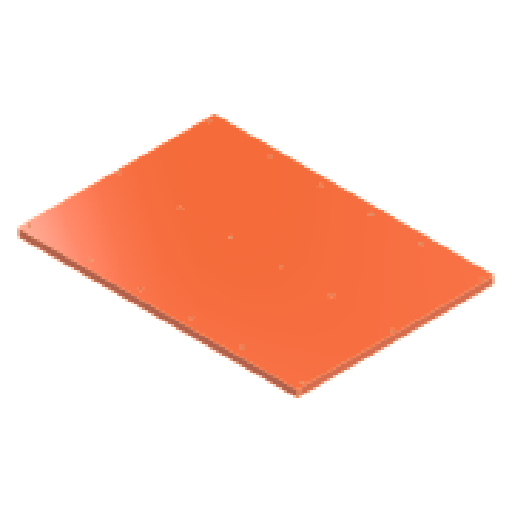
# Autodesk Inventor part: GRJ-04-101A
Saved by Autodesk Inventor 2026.1 (Build 301233000, 233)
## iProperties
Company: Gree
Created: 2025-09-10
Part Number: GRJ-04-101A
Material: Fenolite OR
Document SubType Name: Modeling
Designer: Willian Pinheiro
Density: 1.38 g/cm^3
Appearance: Suave - Laranja claro
Project: GRJ-04
Checked By: Antonio Lucas
Engr Approved By: Antonio Lucas
Description: Base Principal A
Mfg Approved By: Anderson Oliveira
Mass: 1474.18 g
Surface Area: 2294.98 cm^2
Volume: 1068.25 cm^3
Total: 1
Dimensões: 10 x 275 x 390 mm
Author: Willian Pinheiro
Title: Pasta Dissipador G
Revision Number: 00
Autodesk Inventor part; units mm, degrees
ref_plane "YZ Plane" through (0, 0, 0) normal (1, 0, 0) x (0, 1, 0)
ref_plane "XZ Plane" through (0, 0, 0) normal (0, 1, 0) x (-1, 0, 0)
ref_plane "XY Plane" through (0, 0, 0) normal (0, 0, 1) x (1, 0, 0)
sketch "Esboço1" plane through (0, 0, 0) normal (0, 0, 1) x (1, 0, 0)
  line L0 (-195, -137.5) -> (195, -137.5)
  line L1 (195, -137.5) -> (195, 137.5)
  line L2 (195, 137.5) -> (-195, 137.5)
  line L3 (-195, 137.5) -> (-195, -137.5)
  line L4 (190, -137.5) -> (190, 137.5) construction
  line L5 (-273, 0) -> (273, 0) construction
  line L6 (0, -192.5) -> (0, 192.5) construction
  line L7 (-70, 137.5) -> (-70, -137.5) construction
  point P0 (0, 0)
  point P1 (190, 125)
  point P2 (190, 0)
  point P3 (190, -125)
  point P4 (35, 125)
  point P5 (35, 0)
  point P6 (35, -125)
  point P7 (-190, 125)
  point P8 (-190, 0)
  point P9 (-190, -125)
  point P10 (-35, 125)
  point P11 (-35, 0)
  point P12 (-35, -125)
  point P13 (-105, -125)
  point P14 (-105, 0)
  point P15 (-105, 125)
  point P16 (105, 125)
  point P17 (105, 0)
  point P18 (105, -125)
  dimension "d0" = 390
  dimension "d1" = 275
  dimension "d11" = 125
  dimension "d12" = 125
  dimension "d14" = 70
  dimension "d15" = 380
  dimension "d23" = 250
  dimension "d25" = 70
  constraints: 12 end point, 12 symmetric about line, 7 point on line, 3 horizontal alignment, 3 perpendicular, 2 parallel, 2 vertical alignment, 1 horizontal, 1 midpoint, 2 other
  measures "d0" distance of L1.end L2.end
  measures "d1" distance of L2.end L0.start
  measures "d11" distance of point (190, -125) point (190, 0)
  measures "d12" distance of point (190, 125) point (190, 0)
  measures "d14" distance of point (-35, 125) point (35, 125)
  measures "d15" distance of point (-190, 125) point (190, 125)
  measures "d23" distance of point (190, 125) point (190, -125)
  measures "d25" distance of point (-35, 125) point (-105, 125)
extrude "Extrusão1" add sketch "Esboço1" along normal blind 10
hole "Hole2" at (190, 125, 0) at (190, 0, 0) at (190, -125, 0) at (35, 125, 0) at (35, 0, 0) at (35, -125, 0) at (-190, -125, 0) at (-190, 0, 0) at (-190, 125, 0) at (-35, -125, 0) at (-35, 0, 0) at (-35, 125, 0) at (-105, -125, 0) at (-105, 0, 0) at (-105, 125, 0) at (105, 125, 0) at (105, 0, 0) at (105, -125, 0) direction (0, 0, 1) diameter 4.5 end through all countersink diameter 10 countersink angle 90 clearance for "Countersunk Flat Head Hex Socket Screw ISO 10642" size "M4" standard "ISO"
fillet "Fillet1" radius 2 4 edges at (195, 137.5, 5) (195, -137.5, 5) (-195, 137.5, 5) (-195, -137.5, 5)
equation "\"d12\" = d11"
equation "\"d25\" = d14"
